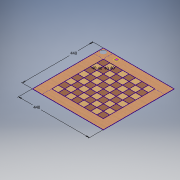
# Autodesk Inventor part: Lid
Saved by Autodesk Inventor 2019 (Build 230136000, 136)
## iProperties
Created: 2019-08-21
Part Number: Lid
Material: Generic
Document SubType Name: Modeling
Designer: Bruno
Density: 1 g/cm^3
Appearance: Default
Author: Bruno
Autodesk Inventor part; units mm, degrees
ref_plane "YZ Plane" through (0, 0, 0) normal (1, 0, 0) x (0, 1, 0)
ref_plane "XZ Plane" through (0, 0, 0) normal (0, 1, 0) x (-1, 0, 0)
ref_plane "XY Plane" through (0, 0, 0) normal (0, 0, 1) x (1, 0, 0)
ref_plane "Work Plane4" through (0, -2, 0) normal (0, -1, 0) x (1, 0, 0)
sketch "Sketch2" plane through (0, -2, 0) normal (0, -1, 0) x (1, 0, 0)
  line L0 (-44.9312, 37.9049) -> (-4.9312, 37.9049)
  line L1 (-4.9312, 37.9049) -> (-4.9312, 77.9049)
  line L2 (-4.9312, 77.9049) -> (-44.9312, 77.9049)
  line L3 (-44.9312, 77.9049) -> (-44.9312, 37.9049)
  line L4 (-4.9312, 117.9049) -> (-44.9312, 117.9049)
  line L5 (-4.9312, 77.9049) -> (-4.9312, 117.9049)
  line L6 (-44.9312, 77.9049) -> (-4.9312, 77.9049)
  line L7 (-44.9312, 117.9049) -> (-44.9312, 77.9049)
  line L8 (-4.9312, 157.9049) -> (-44.9312, 157.9049)
  line L9 (-4.9312, 117.9049) -> (-4.9312, 157.9049)
  line L10 (-44.9312, 117.9049) -> (-4.9312, 117.9049)
  line L11 (-44.9312, 157.9049) -> (-44.9312, 117.9049)
  line L12 (-4.9312, 197.9049) -> (-44.9312, 197.9049)
  line L13 (-4.9312, 157.9049) -> (-4.9312, 197.9049)
  line L14 (-44.9312, 157.9049) -> (-4.9312, 157.9049)
  line L15 (-44.9312, 197.9049) -> (-44.9312, 157.9049)
  line L16 (-4.9312, 237.9049) -> (-44.9312, 237.9049)
  line L17 (-4.9312, 197.9049) -> (-4.9312, 237.9049)
  line L18 (-44.9312, 197.9049) -> (-4.9312, 197.9049)
  line L19 (-44.9312, 237.9049) -> (-44.9312, 197.9049)
  line L20 (-4.9312, 277.9049) -> (-44.9312, 277.9049)
  line L21 (-4.9312, 237.9049) -> (-4.9312, 277.9049)
  line L22 (-44.9312, 237.9049) -> (-4.9312, 237.9049)
  line L23 (-44.9312, 277.9049) -> (-44.9312, 237.9049)
  line L24 (-4.9312, 317.9049) -> (-44.9312, 317.9049)
  line L25 (-4.9312, 277.9049) -> (-4.9312, 317.9049)
  line L26 (-44.9312, 277.9049) -> (-4.9312, 277.9049)
  line L27 (-44.9312, 317.9049) -> (-44.9312, 277.9049)
  line L28 (-4.9312, 357.9049) -> (-44.9312, 357.9049)
  line L29 (-4.9312, 317.9049) -> (-4.9312, 357.9049)
  line L30 (-44.9312, 317.9049) -> (-4.9312, 317.9049)
  line L31 (-44.9312, 357.9049) -> (-44.9312, 317.9049)
  line L32 (35.0688, 77.9049) -> (-4.9312, 77.9049)
  line L33 (35.0688, 37.9049) -> (35.0688, 77.9049)
  line L34 (-4.9312, 37.9049) -> (35.0688, 37.9049)
  line L35 (-4.9312, 77.9049) -> (-4.9312, 37.9049)
  line L36 (35.0688, 117.9049) -> (-4.9312, 117.9049)
  line L37 (35.0688, 77.9049) -> (35.0688, 117.9049)
  line L38 (-4.9312, 77.9049) -> (35.0688, 77.9049)
  line L39 (-4.9312, 117.9049) -> (-4.9312, 77.9049)
  line L40 (35.0688, 157.9049) -> (-4.9312, 157.9049)
  line L41 (35.0688, 117.9049) -> (35.0688, 157.9049)
  line L42 (-4.9312, 117.9049) -> (35.0688, 117.9049)
  line L43 (-4.9312, 157.9049) -> (-4.9312, 117.9049)
  line L44 (35.0688, 197.9049) -> (-4.9312, 197.9049)
  line L45 (35.0688, 157.9049) -> (35.0688, 197.9049)
  line L46 (-4.9312, 157.9049) -> (35.0688, 157.9049)
  line L47 (-4.9312, 197.9049) -> (-4.9312, 157.9049)
  line L48 (35.0688, 237.9049) -> (-4.9312, 237.9049)
  line L49 (35.0688, 197.9049) -> (35.0688, 237.9049)
  line L50 (-4.9312, 197.9049) -> (35.0688, 197.9049)
  line L51 (-4.9312, 237.9049) -> (-4.9312, 197.9049)
  line L52 (35.0688, 277.9049) -> (-4.9312, 277.9049)
  line L53 (35.0688, 237.9049) -> (35.0688, 277.9049)
  line L54 (-4.9312, 237.9049) -> (35.0688, 237.9049)
  line L55 (-4.9312, 277.9049) -> (-4.9312, 237.9049)
  line L56 (35.0688, 317.9049) -> (-4.9312, 317.9049)
  line L57 (35.0688, 277.9049) -> (35.0688, 317.9049)
  line L58 (-4.9312, 277.9049) -> (35.0688, 277.9049)
  line L59 (-4.9312, 317.9049) -> (-4.9312, 277.9049)
  line L60 (35.0688, 357.9049) -> (-4.9312, 357.9049)
  line L61 (35.0688, 317.9049) -> (35.0688, 357.9049)
  line L62 (-4.9312, 317.9049) -> (35.0688, 317.9049)
  line L63 (-4.9312, 357.9049) -> (-4.9312, 317.9049)
  line L64 (75.0688, 77.9049) -> (35.0688, 77.9049)
  line L65 (75.0688, 37.9049) -> (75.0688, 77.9049)
  line L66 (35.0688, 37.9049) -> (75.0688, 37.9049)
  line L67 (35.0688, 77.9049) -> (35.0688, 37.9049)
  line L68 (75.0688, 117.9049) -> (35.0688, 117.9049)
  line L69 (75.0688, 77.9049) -> (75.0688, 117.9049)
  line L70 (35.0688, 77.9049) -> (75.0688, 77.9049)
  line L71 (35.0688, 117.9049) -> (35.0688, 77.9049)
  line L72 (75.0688, 157.9049) -> (35.0688, 157.9049)
  line L73 (75.0688, 117.9049) -> (75.0688, 157.9049)
  line L74 (35.0688, 117.9049) -> (75.0688, 117.9049)
  line L75 (35.0688, 157.9049) -> (35.0688, 117.9049)
  line L76 (75.0688, 197.9049) -> (35.0688, 197.9049)
  line L77 (75.0688, 157.9049) -> (75.0688, 197.9049)
  line L78 (35.0688, 157.9049) -> (75.0688, 157.9049)
  line L79 (35.0688, 197.9049) -> (35.0688, 157.9049)
  line L80 (75.0688, 237.9049) -> (35.0688, 237.9049)
  line L81 (75.0688, 197.9049) -> (75.0688, 237.9049)
  line L82 (35.0688, 197.9049) -> (75.0688, 197.9049)
  line L83 (35.0688, 237.9049) -> (35.0688, 197.9049)
  line L84 (75.0688, 277.9049) -> (35.0688, 277.9049)
  line L85 (75.0688, 237.9049) -> (75.0688, 277.9049)
  line L86 (35.0688, 237.9049) -> (75.0688, 237.9049)
  line L87 (35.0688, 277.9049) -> (35.0688, 237.9049)
  line L88 (75.0688, 317.9049) -> (35.0688, 317.9049)
  line L89 (75.0688, 277.9049) -> (75.0688, 317.9049)
  line L90 (35.0688, 277.9049) -> (75.0688, 277.9049)
  line L91 (35.0688, 317.9049) -> (35.0688, 277.9049)
  line L92 (75.0688, 357.9049) -> (35.0688, 357.9049)
  line L93 (75.0688, 317.9049) -> (75.0688, 357.9049)
  line L94 (35.0688, 317.9049) -> (75.0688, 317.9049)
  line L95 (35.0688, 357.9049) -> (35.0688, 317.9049)
  line L96 (115.0688, 77.9049) -> (75.0688, 77.9049)
  line L97 (115.0688, 37.9049) -> (115.0688, 77.9049)
  line L98 (75.0688, 37.9049) -> (115.0688, 37.9049)
  line L99 (75.0688, 77.9049) -> (75.0688, 37.9049)
  line L100 (115.0688, 117.9049) -> (75.0688, 117.9049)
  line L101 (115.0688, 77.9049) -> (115.0688, 117.9049)
  line L102 (75.0688, 77.9049) -> (115.0688, 77.9049)
  line L103 (75.0688, 117.9049) -> (75.0688, 77.9049)
  line L104 (115.0688, 157.9049) -> (75.0688, 157.9049)
  line L105 (115.0688, 117.9049) -> (115.0688, 157.9049)
  line L106 (75.0688, 117.9049) -> (115.0688, 117.9049)
  line L107 (75.0688, 157.9049) -> (75.0688, 117.9049)
  line L108 (115.0688, 197.9049) -> (75.0688, 197.9049)
  line L109 (115.0688, 157.9049) -> (115.0688, 197.9049)
  line L110 (75.0688, 157.9049) -> (115.0688, 157.9049)
  line L111 (75.0688, 197.9049) -> (75.0688, 157.9049)
  line L112 (115.0688, 237.9049) -> (75.0688, 237.9049)
  line L113 (115.0688, 197.9049) -> (115.0688, 237.9049)
  line L114 (75.0688, 197.9049) -> (115.0688, 197.9049)
  line L115 (75.0688, 237.9049) -> (75.0688, 197.9049)
  line L116 (115.0688, 277.9049) -> (75.0688, 277.9049)
  line L117 (115.0688, 237.9049) -> (115.0688, 277.9049)
  line L118 (75.0688, 237.9049) -> (115.0688, 237.9049)
  line L119 (75.0688, 277.9049) -> (75.0688, 237.9049)
  line L120 (115.0688, 317.9049) -> (75.0688, 317.9049)
  line L121 (115.0688, 277.9049) -> (115.0688, 317.9049)
  line L122 (75.0688, 277.9049) -> (115.0688, 277.9049)
  line L123 (75.0688, 317.9049) -> (75.0688, 277.9049)
  line L124 (115.0688, 357.9049) -> (75.0688, 357.9049)
  line L125 (115.0688, 317.9049) -> (115.0688, 357.9049)
  line L126 (75.0688, 317.9049) -> (115.0688, 317.9049)
  line L127 (75.0688, 357.9049) -> (75.0688, 317.9049)
  line L128 (155.0688, 77.9049) -> (115.0688, 77.9049)
  line L129 (155.0688, 37.9049) -> (155.0688, 77.9049)
  line L130 (115.0688, 37.9049) -> (155.0688, 37.9049)
  line L131 (115.0688, 77.9049) -> (115.0688, 37.9049)
  line L132 (155.0688, 117.9049) -> (115.0688, 117.9049)
  line L133 (155.0688, 77.9049) -> (155.0688, 117.9049)
  line L134 (115.0688, 77.9049) -> (155.0688, 77.9049)
  line L135 (115.0688, 117.9049) -> (115.0688, 77.9049)
  line L136 (155.0688, 157.9049) -> (115.0688, 157.9049)
  line L137 (155.0688, 117.9049) -> (155.0688, 157.9049)
  line L138 (115.0688, 117.9049) -> (155.0688, 117.9049)
  line L139 (115.0688, 157.9049) -> (115.0688, 117.9049)
  line L140 (155.0688, 197.9049) -> (115.0688, 197.9049)
  line L141 (155.0688, 157.9049) -> (155.0688, 197.9049)
  line L142 (115.0688, 157.9049) -> (155.0688, 157.9049)
  line L143 (115.0688, 197.9049) -> (115.0688, 157.9049)
  line L144 (155.0688, 237.9049) -> (115.0688, 237.9049)
  line L145 (155.0688, 197.9049) -> (155.0688, 237.9049)
  line L146 (115.0688, 197.9049) -> (155.0688, 197.9049)
  line L147 (115.0688, 237.9049) -> (115.0688, 197.9049)
  line L148 (155.0688, 277.9049) -> (115.0688, 277.9049)
  line L149 (155.0688, 237.9049) -> (155.0688, 277.9049)
  line L150 (115.0688, 237.9049) -> (155.0688, 237.9049)
  line L151 (115.0688, 277.9049) -> (115.0688, 237.9049)
  line L152 (155.0688, 317.9049) -> (115.0688, 317.9049)
  line L153 (155.0688, 277.9049) -> (155.0688, 317.9049)
  line L154 (115.0688, 277.9049) -> (155.0688, 277.9049)
  line L155 (115.0688, 317.9049) -> (115.0688, 277.9049)
  line L156 (155.0688, 357.9049) -> (115.0688, 357.9049)
  line L157 (155.0688, 317.9049) -> (155.0688, 357.9049)
  line L158 (115.0688, 317.9049) -> (155.0688, 317.9049)
  line L159 (115.0688, 357.9049) -> (115.0688, 317.9049)
  line L160 (195.0688, 77.9049) -> (155.0688, 77.9049)
  line L161 (195.0688, 37.9049) -> (195.0688, 77.9049)
  line L162 (155.0688, 37.9049) -> (195.0688, 37.9049)
  line L163 (155.0688, 77.9049) -> (155.0688, 37.9049)
  line L164 (195.0688, 117.9049) -> (155.0688, 117.9049)
  line L165 (195.0688, 77.9049) -> (195.0688, 117.9049)
  line L166 (155.0688, 77.9049) -> (195.0688, 77.9049)
  line L167 (155.0688, 117.9049) -> (155.0688, 77.9049)
  line L168 (195.0688, 157.9049) -> (155.0688, 157.9049)
  line L169 (195.0688, 117.9049) -> (195.0688, 157.9049)
  line L170 (155.0688, 117.9049) -> (195.0688, 117.9049)
  line L171 (155.0688, 157.9049) -> (155.0688, 117.9049)
  line L172 (195.0688, 197.9049) -> (155.0688, 197.9049)
  line L173 (195.0688, 157.9049) -> (195.0688, 197.9049)
  line L174 (155.0688, 157.9049) -> (195.0688, 157.9049)
  line L175 (155.0688, 197.9049) -> (155.0688, 157.9049)
  line L176 (195.0688, 237.9049) -> (155.0688, 237.9049)
  line L177 (195.0688, 197.9049) -> (195.0688, 237.9049)
  line L178 (155.0688, 197.9049) -> (195.0688, 197.9049)
  line L179 (155.0688, 237.9049) -> (155.0688, 197.9049)
  line L180 (195.0688, 277.9049) -> (155.0688, 277.9049)
  line L181 (195.0688, 237.9049) -> (195.0688, 277.9049)
  line L182 (155.0688, 237.9049) -> (195.0688, 237.9049)
  line L183 (155.0688, 277.9049) -> (155.0688, 237.9049)
  line L184 (195.0688, 317.9049) -> (155.0688, 317.9049)
  line L185 (195.0688, 277.9049) -> (195.0688, 317.9049)
  line L186 (155.0688, 277.9049) -> (195.0688, 277.9049)
  line L187 (155.0688, 317.9049) -> (155.0688, 277.9049)
  line L188 (195.0688, 357.9049) -> (155.0688, 357.9049)
  line L189 (195.0688, 317.9049) -> (195.0688, 357.9049)
  line L190 (155.0688, 317.9049) -> (195.0688, 317.9049)
  line L191 (155.0688, 357.9049) -> (155.0688, 317.9049)
  line L192 (235.0688, 77.9049) -> (195.0688, 77.9049)
  line L193 (235.0688, 37.9049) -> (235.0688, 77.9049)
  line L194 (195.0688, 37.9049) -> (235.0688, 37.9049)
  line L195 (195.0688, 77.9049) -> (195.0688, 37.9049)
  line L196 (235.0688, 117.9049) -> (195.0688, 117.9049)
  line L197 (235.0688, 77.9049) -> (235.0688, 117.9049)
  line L198 (195.0688, 77.9049) -> (235.0688, 77.9049)
  line L199 (195.0688, 117.9049) -> (195.0688, 77.9049)
  line L200 (235.0688, 157.9049) -> (195.0688, 157.9049)
  line L201 (235.0688, 117.9049) -> (235.0688, 157.9049)
  line L202 (195.0688, 117.9049) -> (235.0688, 117.9049)
  line L203 (195.0688, 157.9049) -> (195.0688, 117.9049)
  line L204 (235.0688, 197.9049) -> (195.0688, 197.9049)
  line L205 (235.0688, 157.9049) -> (235.0688, 197.9049)
  line L206 (195.0688, 157.9049) -> (235.0688, 157.9049)
  line L207 (195.0688, 197.9049) -> (195.0688, 157.9049)
  line L208 (235.0688, 237.9049) -> (195.0688, 237.9049)
  line L209 (235.0688, 197.9049) -> (235.0688, 237.9049)
  line L210 (195.0688, 197.9049) -> (235.0688, 197.9049)
  line L211 (195.0688, 237.9049) -> (195.0688, 197.9049)
  line L212 (235.0688, 277.9049) -> (195.0688, 277.9049)
  line L213 (235.0688, 237.9049) -> (235.0688, 277.9049)
  line L214 (195.0688, 237.9049) -> (235.0688, 237.9049)
  line L215 (195.0688, 277.9049) -> (195.0688, 237.9049)
  line L216 (235.0688, 317.9049) -> (195.0688, 317.9049)
  line L217 (235.0688, 277.9049) -> (235.0688, 317.9049)
  line L218 (195.0688, 277.9049) -> (235.0688, 277.9049)
  line L219 (195.0688, 317.9049) -> (195.0688, 277.9049)
  line L220 (235.0688, 357.9049) -> (195.0688, 357.9049)
  line L221 (235.0688, 317.9049) -> (235.0688, 357.9049)
  line L222 (195.0688, 317.9049) -> (235.0688, 317.9049)
  line L223 (195.0688, 357.9049) -> (195.0688, 317.9049)
  line L224 (275.0688, 77.9049) -> (235.0688, 77.9049)
  line L225 (275.0688, 37.9049) -> (275.0688, 77.9049)
  line L226 (235.0688, 37.9049) -> (275.0688, 37.9049)
  line L227 (235.0688, 77.9049) -> (235.0688, 37.9049)
  line L228 (275.0688, 117.9049) -> (235.0688, 117.9049)
  line L229 (275.0688, 77.9049) -> (275.0688, 117.9049)
  line L230 (235.0688, 77.9049) -> (275.0688, 77.9049)
  line L231 (235.0688, 117.9049) -> (235.0688, 77.9049)
  line L232 (275.0688, 157.9049) -> (235.0688, 157.9049)
  line L233 (275.0688, 117.9049) -> (275.0688, 157.9049)
  line L234 (235.0688, 117.9049) -> (275.0688, 117.9049)
  line L235 (235.0688, 157.9049) -> (235.0688, 117.9049)
  line L236 (275.0688, 197.9049) -> (235.0688, 197.9049)
  line L237 (275.0688, 157.9049) -> (275.0688, 197.9049)
  line L238 (235.0688, 157.9049) -> (275.0688, 157.9049)
  line L239 (235.0688, 197.9049) -> (235.0688, 157.9049)
  line L240 (275.0688, 237.9049) -> (235.0688, 237.9049)
  line L241 (275.0688, 197.9049) -> (275.0688, 237.9049)
  line L242 (235.0688, 197.9049) -> (275.0688, 197.9049)
  line L243 (235.0688, 237.9049) -> (235.0688, 197.9049)
  line L244 (275.0688, 277.9049) -> (235.0688, 277.9049)
  line L245 (275.0688, 237.9049) -> (275.0688, 277.9049)
  line L246 (235.0688, 237.9049) -> (275.0688, 237.9049)
  line L247 (235.0688, 277.9049) -> (235.0688, 237.9049)
  line L248 (275.0688, 317.9049) -> (235.0688, 317.9049)
  line L249 (275.0688, 277.9049) -> (275.0688, 317.9049)
  line L250 (235.0688, 277.9049) -> (275.0688, 277.9049)
  line L251 (235.0688, 317.9049) -> (235.0688, 277.9049)
  line L252 (275.0688, 357.9049) -> (235.0688, 357.9049)
  line L253 (275.0688, 317.9049) -> (275.0688, 357.9049)
  line L254 (235.0688, 317.9049) -> (275.0688, 317.9049)
  line L255 (235.0688, 357.9049) -> (235.0688, 317.9049)
  line L256 (-104.9312, -22.0951) -> (-104.9312, 417.9049)
  line L257 (-104.9312, 417.9049) -> (335.0688, 417.9049)
  line L258 (335.0688, 417.9049) -> (335.0688, -22.0951)
  line L259 (335.0688, -22.0951) -> (-104.9312, -22.0951)
  line L260 (-44.9312, 357.9049) -> (-44.9312, 417.9049) construction
  line L261 (-44.9312, 37.9049) -> (-44.9312, -22.0951) construction
  line L262 (-44.9312, 37.9049) -> (-104.9312, 37.9049) construction
  line L263 (275.0688, 37.9049) -> (335.0688, 37.9049) construction
  point P0 (0, 0)
  dimension "d4" = 40
  dimension "d5" = 40
  dimension "d8" = 40
  dimension "d11" = 40
  dimension "d14" = 440
  dimension "d15" = 440
  constraints: 528 end point, 7 perpendicular, 4 collinear, 4 point on line, 4 vertical, 3 horizontal, 2 parallel, 502 other
  measures "d4" distance of L2.end L1.end
  measures "d5" distance of L1.end L0.end
  measures "d8" distance of L1.end L4.start
  measures "d11" distance of L1.end L32.start
  measures "d14" distance of L256.end L257.end
  measures "d15" distance of L256.start L256.end
extrude "Extrusion2" add sketch "Sketch2" along normal blind 3
extrude "Extrusion3" add sketch "Sketch2" along normal blind 2 separate body contours L1 L32 L33 L34 | L7 L4 L5 L2 | L9 L40 L41 L36 | L37 L68 L69 L64 | L65 L96 L97 L98 | L15 L12 L13 L8 | L17 L48 L49 L44 | L45 L76 L77 L72 | L73 L104 L105 L100 | L101 L132 L133 L128 | L129 L160 L161 L162 | L23 L20 L21 L16 | L25 L56 L57 L52 | L53 L84 L85 L80 | L81 L112 L113 L108 | L109 L140 L141 L136 | L137 L168 L169 L164 | L165 L196 L197 L192 | L193 L224 L225 L226 | L31 L28 L29 L24 | L61 L92 L93 L88 | L89 L120 L121 L116 | L117 L148 L149 L144 | L145 L176 L177 L172 | L173 L204 L205 L200 | L201 L232 L233 L228 | L125 L156 L157 L152 | L153 L184 L185 L180 | L181 L212 L213 L208 | L209 L240 L241 L236 | L189 L220 L221 L216 | L217 L248 L249 L244
extrude "Extrusion4" add sketch "Sketch2" along normal blind 2 separate body contours L3 L2 L1 L0 | L5 L36 L37 L32 | L33 L64 L65 L66 | L11 L8 L9 L4 | L13 L44 L45 L40 | L41 L72 L73 L68 | L69 L100 L101 L96 | L97 L128 L129 L130 | L19 L16 L17 L12 | L21 L52 L53 L48 | L49 L80 L81 L76 | L77 L108 L109 L104 | L105 L136 L137 L132 | L133 L164 L165 L160 | L161 L192 L193 L194 | L27 L24 L25 L20 | L29 L60 L61 L56 | L57 L88 L89 L84 | L85 L116 L117 L112 | L113 L144 L145 L140 | L141 L172 L173 L168 | L169 L200 L201 L196 | L197 L228 L229 L224 | L93 L124 L125 L120 | L121 L152 L153 L148 | L149 L180 L181 L176 | L177 L208 L209 L204 | L205 L236 L237 L232 | L157 L188 L189 L184 | L185 L216 L217 L212 | L213 L244 L245 L240 | L221 L252 L253 L248
sketch "Sketch3" plane through (0, -2, 0) normal (0, 1, 0) x (1, 0, 0)
  circle A0 centre (-14.9312, 4.5951) radius 12.5
  line L0 (-104.9312, 22.0951) -> (-104.9312, -417.9049) projected
  line L1 (-104.9312, -417.9049) -> (335.0688, -417.9049) projected
  line L2 (335.0688, 22.0951) -> (-104.9312, 22.0951) projected
  line L3 (335.0688, -417.9049) -> (335.0688, 22.0951) projected
  point P0 (0, 0)
  dimension "d22" = 25
  dimension "d32" = 350
  dimension "d34" = 17.5
  constraints: 1 centre point
  measures "d22" diameter of A0
  measures "d32" distance from line of L3 A0.centre
  measures "d34" distance from line of L2 A0.centre
extrude "Extrusion5" cut sketch "Sketch3" against normal up to next contours A0 bodies 1
sketch "Sketch4" plane through (0, -2, 0) normal (0, 1, 0) x (1, 0, 0)
  circle A0 centre (-94.9312, 12.0951) radius 2.625
  line L0 (-104.9312, 22.0951) -> (-104.9312, -417.9049) projected
  line L1 (335.0688, 22.0951) -> (-104.9312, 22.0951) projected
  circle A1 centre (325.0688, 12.0951) radius 2.625
  circle A2 centre (325.0688, -407.9049) radius 2.625
  circle A3 centre (-94.9312, -407.9049) radius 2.625
  line L2 (325.0688, 12.0951) -> (325.0688, 22.0951) construction
  line L3 (325.0688, 12.0951) -> (335.0688, 12.0951) construction
  line L4 (335.0688, -417.9049) -> (335.0688, 22.0951) projected
  line L5 (-104.9312, -407.9049) -> (-94.9312, -407.9049) construction
  line L6 (-94.9312, -407.9049) -> (-94.9312, -417.9049) construction
  line L7 (-104.9312, -417.9049) -> (335.0688, -417.9049) projected
  line L8 (325.0688, -407.9049) -> (325.0688, -417.9049) construction
  line L9 (325.0688, -407.9049) -> (335.0688, -407.9049) construction
  line L10 (-94.9312, 12.0951) -> (-94.9312, 22.0951) construction
  point P0 (0, 0)
  dimension "d35" = 5.25
  dimension "d37" = 10
  dimension "d38" = 5.25
  dimension "d39" = 5.25
  dimension "d40" = 5.25
  constraints: 14 end point, 8 point on line, 6 equal length, 4 centre point, 4 perpendicular, 1 horizontal, 1 parallel
  measures "d35" diameter of A0
  measures "d37" distance from line of L1 L10.start
  measures "d38" diameter of A1
  measures "d39" diameter of A2
  measures "d40" diameter of A3
extrude "Extrusion6" cut sketch "Sketch4" against normal up to next contours A0 | A1 | A2 | A3 bodies 1
body "Solid2"
body "Solid3"
body "Solid4"
